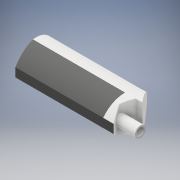
# Autodesk Inventor part: Sci-Fi Raycasting weapon F
Saved by Autodesk Inventor 2017 (Build 210142000, 142)
## iProperties
Created: 2019-09-03
Part Number: Sci-Fi Raycasting weapon F
Material: Generic
Document SubType Name: Modeling
Designer: Victor
Density: 1 g/cm^3
Appearance: Default
Author: Victor
Autodesk Inventor part; units mm, degrees
ref_plane "YZ Plane" through (0, 0, 0) normal (1, 0, 0) x (0, 1, 0)
ref_plane "XZ Plane" through (0, 0, 0) normal (0, 1, 0) x (-1, 0, 0)
ref_plane "XY Plane" through (0, 0, 0) normal (0, 0, 1) x (1, 0, 0)
sketch "Sketch1" plane through (0, 0, 0) normal (0, 0, 1) x (1, 0, 0)
  line L0 (0, 0) -> (0, 5)
  line L1 (0, 5) -> (-22, 5)
  line L2 (0, 0) -> (-22, 0)
  line L3 (-22, 5) -> (-22, 0)
  dimension "d0" = 5
  dimension "d3" = 22
  dimension "d4" = 22
  constraints: 8 end point, 2 horizontal, 1 vertical
  measures "d0" distance of L0.start L0.end
  measures "d3" distance of L0.end L1.end
  measures "d4" distance of L0.start L2.end
extrude "Extrusion1" add sketch "Sketch1" along normal blind 7
sketch "Sketch2" plane through (0, 0, 0) normal (1, 0, 0) x (0, 0, -1)
  line L0 (-7, 0) -> (-7, 5) projected
  line L1 (0, 5) -> (-7, 5) projected
  line L2 (0, 0) -> (0, 5) projected
  line L3 (-4.5, 5) -> (-7, 5)
  line L4 (-7, 5) -> (-7, 0)
  line L5 (0, 0) -> (0, 5)
  line L6 (0, 5) -> (-2.5, 5)
  arc A0 (-4.5, 5) -> (-7, 0) centre (0.2327, -0.4914) ccw
  arc A1 (0, 0) -> (-2.5, 5) centre (-7.2331, -0.4916) ccw
  dimension "d11" = 4.5
  dimension "d12" = 2.5
  dimension "d13" = 0
  constraints: 8 end point, 4 point on circle, 3 coincident, 2 centre point, 1 horizontal alignment, 1 vertical
  measures "d11" distance of L1.start L3.start
  measures "d12" distance of L1.start L6.end
  measures "d13" vertical distance of L1.start L6.end
extrude "Extrusion2" cut sketch "Sketch2" against normal blind 30
sketch "Sketch4" plane through (-22, 0, 0) normal (0, -1, 0) x (1, 0, 0)
  line L0 (0, 0) -> (0, 7) projected
  line L1 (0, 7) -> (22, 7)
  line L2 (22, 7) -> (22, 0)
  line L3 (22, 0) -> (0, 0)
  line L4 (0, 0) -> (0, 7)
  constraints: 8 end point, 2 parallel, 1 horizontal, 1 perpendicular
extrude "Extrusion5" add sketch "Sketch4" along normal blind 5
sketch "Sketch5" plane through (0, 5, 4.5) normal (1, 0, 0) x (0, 0, -1)
  line L0 (-2.5, -10) -> (4.5, -10) projected
  line L1 (0, -10) -> (-2.5, -10)
  line L2 (2, -10) -> (4.5, -10)
  line L3 (-2.5, -5) -> (-2.5, -10) projected
  arc A0 (-2.5, -5) -> (0, -10) centre (4.7329, -4.5086) ccw
  arc A1 (2, -10) -> (4.5, -5) centre (-2.7331, -4.5085) ccw
  line L4 (-2.5, -10) -> (-2.5, -5)
  line L5 (4.5, -10) -> (4.5, -4.0169)
  line L6 (4.5, -5) -> (4.5, -10) projected
  dimension "d22" = 4.5
  dimension "d23" = 2.5
  dimension "d24" = 5
  dimension "d25" = 5
  constraints: 8 end point, 5 point on circle, 2 centre point, 1 collinear
  measures "d22" horizontal distance of L6.start L1.start
  measures "d23" horizontal distance of L6.start L2.start
  measures "d24" vertical distance of L1.start L6.start
  measures "d25" vertical distance of L6.start L2.start
extrude "Extrusion6" cut sketch "Sketch5" against normal blind 22
sketch "Sketch6" plane through (0, 0, 0) normal (0, 0, 1) x (1, 0, 0)
  line L0 (-22, 0) -> (-22, -5) projected
  line L1 (-22, -5) -> (-22, 5)
  line L2 (-22, -5) -> (-20, -5)
  line L3 (-22, -5) -> (0, -5) projected
  line L4 (-20, -5) -> (-22, 5)
  point P0 (0, 0)
  dimension "d28" = 2
  constraints: 6 end point, 1 collinear, 1 point on line
  measures "d28" distance of L0.end L2.end
extrude "Extrusion7" cut sketch "Sketch6" along normal blind 22
sketch "Sketch7" plane through (0, 5, 4.5) normal (1, 0, 0) x (0, 0, -1)
  line L0 (2, 0) -> (0, 0) projected
  line L1 (0, 0) -> (2, 0)
  arc A0 (2, -10) -> (4.5, -5) centre (-2.7331, -4.5085) ccw projected
  line L2 (2, -10) -> (0, -10) projected
  line L3 (2, -10) -> (0, -10)
  arc A1 (0, 0) -> (-2.5, -5) centre (4.7327, -5.4914) ccw projected
  arc A2 (0, 0) -> (0, -10) centre (3.75, -5) ccw
  arc A3 (4.5, -5) -> (2, 0) centre (-2.7331, -5.4916) ccw projected
  arc A4 (2, -10) -> (2, 0) centre (-1.75, -5) ccw
  constraints: 6 point on circle, 4 end point, 2 centre point, 1 collinear, 1 horizontal
extrude "Extrusion8" add sketch "Sketch7" along normal blind 5
sketch "Sketch11" plane through (0, 0, 0) normal (0, 0, 1) x (1, 0, 0)
  line L0 (5, -5) -> (5, 5) projected
  line L1 (0, 0) -> (0, 5) projected
  line L2 (0, 5) -> (3.9, 0)
  line L3 (3.9, 0) -> (2.4, 0)
  line L4 (2.4, 0) -> (1.1568, -2.5)
  line L5 (1.1568, -2.5) -> (2.4, -5)
  line L6 (0, -5) -> (5, -5) projected
  line L7 (2.4, -5) -> (5, -5)
  line L8 (5, 0) -> (5, -5)
  line L9 (5, 0) -> (3.9, 0)
  line L10 (0, 5) -> (5, 5) projected
  line L11 (5, 0) -> (5, 5)
  line L12 (5, 5) -> (0, 5)
  dimension "d50" = 3.9
  dimension "d51" = 5
  dimension "d52" = 1.5
  dimension "d53" = 5
  dimension "d54" = 2.5
  dimension "d55" = 127.119
  dimension "d56" = 2.328
  constraints: 18 end point, 2 perpendicular, 2 vertical, 1 collinear, 1 midpoint, 1 point on line
  measures "d50" distance of L1.start L2.end
  measures "d51" distance from line of L0 L1.start
  measures "d52" distance of L2.end L3.end
  measures "d53" vertical distance of L1.end L2.end
  measures "d54" vertical distance of L3.end L4.end
  measures "d55" angle of L5 L4
  measures "d56" distance from line of L0.start L5
extrude "Extrusion12" cut sketch "Sketch11" along normal blind 10
sketch "Sketch12" plane through (0, 0, 0) normal (1, 0, 0) x (0, 1, 0)
  line L0 (-2.5, 0.5218) -> (-2.5, 6.4782) projected
  circle A0 centre (-2.5, 3.5) radius 1.25
  point P0 (0, 0)
  dimension "d59" = 2.5
  constraints: 1 centre point, 1 midpoint
  measures "d59" diameter of A0
extrude "Extrusion13" add sketch "Sketch12" along normal blind 6
sketch "Sketch13" plane through (6, -2.5, 3.5) normal (1, 0, 0) x (0, 0, -1)
  circle A0 centre (0, 0) radius 0.875
  point P0 (3.5, 2.5)
  dimension "d62" = 1.75
  constraints: 1 centre point
  measures "d62" diameter of A0
extrude "Extrusion14" cut sketch "Sketch13" against normal blind 6
equation "\"d25\" = d24"
body "Solid1"
